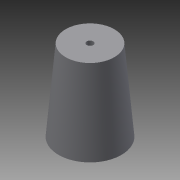
# Autodesk Inventor part: brush fitting parta v4
Saved by Autodesk Inventor 2013 SP2 (Build 170200200, 200)
## iProperties
Created: 2017-05-15
Part Number: brush fitting parta v4
Material: Generic
Document SubType Name: Modeling
Designer: Herman de Vries
Density: 1 g/cm^3
Author: Herman de Vries
Autodesk Inventor part; units mm, degrees
ref_plane "YZ Plane" through (0, 0, 0) normal (1, 0, 0) x (0, 1, 0)
ref_plane "XZ Plane" through (0, 0, 0) normal (0, 1, 0) x (-1, 0, 0)
ref_plane "XY Plane" through (0, 0, 0) normal (0, 0, 1) x (1, 0, 0)
sketch "Sketch1" plane through (0, 0, 0) normal (1, 0, 0) x (0, 1, 0)
  line L0 (0, 20) -> (6, 20) construction
  arc A0 (7.7498, 0) -> (6, 20) centre (-30.6677, 6.7154) ccw construction
  line L1 (0, 16) -> (0, 0) construction
  line L2 (6, 20) -> (2.4961, 20) construction
  line L3 (7.7498, 0) -> (4.5, 0) construction
  line L4 (4.5, 10) -> (0, 10)
  line L5 (4.5, 10) -> (4.5, 0)
  line L6 (0, 16) -> (0, 10)
  line L7 (7.7498, 0) -> (6, 20) construction
  line L8 (4.5, 0) -> (7.7498, 0)
  line L9 (7.7498, 0) -> (6, 20)
  line L10 (0, 16) -> (0.8, 16)
  line L11 (0.8, 16) -> (0.8, 20)
  line L12 (0.8, 20) -> (6, 20)
  dimension "d0" = 6
  dimension "d5" = 4.5
  dimension "d11" = 10
  dimension "d12" = 20
  dimension "d13" = 95
  dimension "d21" = 4
  dimension "d22" = 0.8
  constraints: 26 end point, 3 collinear, 3 horizontal, 2 parallel, 2 perpendicular, 2 point on circle, 1 centre point, 1 horizontal alignment, 1 point on line, 1 vertical, 1 vertical alignment
  measures "d0" distance of L0.start L0.end
  measures "d5" distance of L4.start L4.end
  measures "d11" distance from line of L4 L1.end
  measures "d12" distance from line of L0 L1.end
  measures "d13" angle of L3 L7
  measures "d21" distance of L10.end L11.end
  measures "d22" distance of L1.start L10.end
revolve "Revolution1" add sketch "Sketch1" angle 360 about axis through (0, 0, 16) along (0, 0, -1)
body "Solid1"
